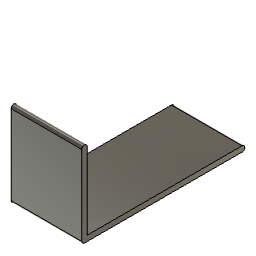
Nintendo 64 Bookends (Autodesk Fusion 360 design; units mm, degrees)
Autodesk Fusion 360 part; units mm, degrees
sketch "Sketch1" plane through (0, 0, 0) normal (0, 0, 1) x (1, 0, 0)
  line L0 (0, 0) -> (39, 0)
  line L1 (39, 0) -> (39, 87)
  line L2 (39, 87) -> (0, 87)
  line L3 (0, 87) -> (0, 0)
  line L4 (0, 0) -> (39, 0)
  line L5 (39, 0) -> (39, -3)
  line L6 (39, -3) -> (0, -3)
  line L7 (0, -3) -> (0, 0)
  dimension "d1" = 39
  dimension "d2" = 87
  dimension "d3" = 3
  constraint horizontal L0
  constraint vertical L1
  constraint horizontal L2
  constraint vertical L3
  constraint coincident L0.start L3.end
  constraint horizontal L4
  constraint vertical L5
  constraint horizontal L6
  constraint vertical L7
  measures "d1" distance of L0.start L0.end
  measures "d2" distance of L0.start L2.end
  measures "d3" distance of L0.start L6.end
extrude "Extrude1" add sketch "Sketch1" along normal blind 47 contours L0 L4 L5 L6 L7
extrude "Extrude2" add sketch "Sketch1" along normal blind 3 contours L0 L1 L2 L3 L4
fillet "Fillet1" radius 1.5 3 edges at (19.5, 87, 3) (19.5, 0, 47) (19.5, -3, 47)
fillet "Fillet2" radius 1.5 2 edges at (19.5, -3, 0) (19.5, 87, 0)
sketch "Sketch2" plane through (0, 0, 0) normal (0, 0, -1) x (1, 0, 0)
  line L0 (0, -85.5) -> (39, -85.5)
  line L1 (39, -85.5) -> (39, 1.5)
  line L2 (39, 1.5) -> (0, 1.5)
  line L3 (0, 1.5) -> (0, -85.5)
  line L4 (30.9966, -51.6762) -> (29.7025, -51.6762)
  line L5 (29.7025, -51.6762) -> (29.7025, -54.5517)
  line L6 (29.7025, -54.5517) -> (30.5781, -54.5517)
  line L7 (30.5781, -54.5517) -> (30.5781, -52.9028)
  line L8 (30.5781, -52.9028) -> (30.5856, -52.9028)
  line L9 (30.5856, -52.9028) -> (31.1629, -54.5517)
  line L10 (31.1629, -54.5517) -> (32.4569, -54.5517)
  line L11 (32.4569, -54.5517) -> (32.4569, -51.6762)
  line L12 (32.4569, -51.6762) -> (31.5818, -51.6762)
  line L13 (31.5818, -51.6762) -> (31.5818, -53.336)
  line L14 (31.5818, -53.336) -> (31.574, -53.336)
  line L15 (31.574, -53.336) -> (30.9966, -51.6762)
  line L16 (26.1146, -51.6762) -> (24.8204, -51.6762)
  line L17 (24.8204, -51.6762) -> (24.8204, -54.5517)
  line L18 (24.8204, -54.5517) -> (25.6956, -54.5517)
  line L19 (25.6956, -54.5517) -> (25.6956, -52.9028)
  line L20 (25.6956, -52.9028) -> (25.7034, -52.9028)
  line L21 (25.7034, -52.9028) -> (26.2807, -54.5517)
  line L22 (26.2807, -54.5517) -> (27.5748, -54.5517)
  line L23 (27.5748, -54.5517) -> (27.5748, -51.6762)
  line L24 (27.5748, -51.6762) -> (26.6994, -51.6762)
  line L25 (26.6994, -51.6762) -> (26.6994, -53.336)
  line L26 (26.6994, -53.336) -> (26.6918, -53.336)
  line L27 (26.6918, -53.336) -> (26.1146, -51.6762)
  line L28 (17.7082, -51.6762) -> (16.414, -51.6762)
  line L29 (16.414, -51.6762) -> (16.414, -54.5517)
  line L30 (16.414, -54.5517) -> (17.2893, -54.5517)
  line L31 (17.2893, -54.5517) -> (17.2893, -52.9028)
  line L32 (17.2893, -52.9028) -> (17.2972, -52.9028)
  line L33 (17.2972, -52.9028) -> (17.8744, -54.5517)
  line L34 (17.8744, -54.5517) -> (19.1685, -54.5517)
  line L35 (19.1685, -54.5517) -> (19.1685, -51.6762)
  line L36 (19.1685, -51.6762) -> (18.2934, -51.6762)
  line L37 (18.2934, -51.6762) -> (18.2934, -53.336)
  line L38 (18.2934, -53.336) -> (18.2857, -53.336)
  line L39 (18.2857, -53.336) -> (17.7082, -51.6762)
  line L40 (29.1739, -54.5517) -> (28.0946, -54.5517)
  line L41 (28.0946, -54.5517) -> (28.0946, -51.6762)
  line L42 (28.0946, -51.6762) -> (29.1739, -51.6762)
  line L43 (29.1739, -51.6762) -> (29.1739, -54.5517)
  line L44 (23.8216, -53.7705) -> (24.5075, -53.7705)
  line L45 (24.5075, -53.7705) -> (24.5075, -54.5517)
  line L46 (24.5075, -54.5517) -> (22.0544, -54.5517)
  line L47 (22.0544, -54.5517) -> (22.0544, -53.7705)
  line L48 (22.0544, -53.7705) -> (22.7426, -53.7705)
  line L49 (22.7426, -53.7705) -> (22.7426, -51.6762)
  line L50 (22.7426, -51.6762) -> (23.8216, -51.6762)
  line L51 (23.8216, -51.6762) -> (23.8216, -53.7705)
  line L52 (21.7356, -54.5524) -> (19.601, -54.5524)
  line L53 (19.601, -54.5524) -> (19.601, -53.7919)
  line L54 (19.601, -53.7919) -> (20.6733, -53.7919)
  line L55 (20.6733, -53.7919) -> (20.6733, -53.4911)
  line L56 (20.6733, -53.4911) -> (19.6859, -53.4911)
  line L57 (19.6859, -53.4911) -> (19.6859, -52.754)
  line L58 (19.6859, -52.754) -> (20.6733, -52.754)
  line L59 (20.6733, -52.754) -> (20.6733, -52.4313)
  line L60 (20.6733, -52.4313) -> (19.5669, -52.4313)
  line L61 (19.5669, -52.4313) -> (19.5669, -51.677)
  line L62 (19.5669, -51.677) -> (21.7356, -51.677)
  line L63 (21.7356, -51.677) -> (21.7356, -54.5524)
  line L64 (19.9291, -48.5819) -> (22.2174, -44.4981)
  line L65 (22.2174, -44.4981) -> (19.9291, -45.375)
  line L66 (19.9291, -45.375) -> (17.745, -44.5387)
  line L67 (17.745, -44.5387) -> (17.16, -45.1951)
  line L68 (17.16, -45.1951) -> (17.16, -49.6558)
  line L69 (17.16, -49.6558) -> (19.9291, -48.5819)
  line L70 (12.8202, -33.9096) -> (16.9532, -39.3035)
  line L71 (16.9532, -39.3035) -> (16.9532, -32.172)
  line L72 (16.9532, -32.172) -> (19.9292, -30.9133)
  line L73 (19.9292, -30.9133) -> (19.9292, -43.0951)
  line L74 (19.9292, -43.0951) -> (16.9532, -44.2347)
  line L75 (16.9532, -44.2347) -> (12.8202, -38.3275)
  line L76 (12.8202, -38.3275) -> (12.8202, -45.838)
  line L77 (12.8202, -45.838) -> (10.0098, -46.9218)
  line L78 (10.0098, -46.9218) -> (10.0098, -35.0899)
  line L79 (10.0098, -35.0899) -> (12.8202, -33.9096)
  line L80 (27.038, -33.9096) -> (24.4011, -35.0771)
  line L81 (24.4011, -35.0771) -> (27.038, -40.1964)
  line L82 (27.038, -40.1964) -> (27.038, -33.9096)
  line L83 (24.2275, -46.9219) -> (22.9048, -44.2351)
  line L84 (22.9048, -44.2351) -> (22.2174, -44.4981)
  line L85 (22.2174, -44.4981) -> (19.9291, -48.5819)
  line L86 (19.9291, -48.5819) -> (22.6984, -49.6589)
  line L87 (22.6984, -49.6589) -> (24.2275, -46.9219)
  line L88 (17.745, -44.5387) -> (15.6298, -46.9219)
  line L89 (15.6298, -46.9219) -> (12.8202, -45.838)
  line L90 (12.8202, -45.838) -> (12.8202, -38.3275)
  line L91 (12.8202, -38.3275) -> (16.9532, -44.2347)
  line L92 (16.9532, -44.2347) -> (17.745, -44.5387)
  line L93 (27.038, -45.8381) -> (29.8484, -46.9219)
  line L94 (29.8484, -46.9219) -> (29.8484, -35.09)
  line L95 (29.8484, -35.09) -> (27.038, -33.9096)
  line L96 (27.038, -33.9096) -> (27.038, -40.1964)
  line L97 (27.038, -40.1964) -> (22.9048, -32.1719)
  line L98 (22.9048, -32.1719) -> (19.9292, -30.9133)
  line L99 (19.9292, -30.9133) -> (19.9292, -43.0951)
  line L100 (19.9292, -43.0951) -> (22.9048, -44.2351)
  line L101 (22.9048, -44.2351) -> (22.9048, -38.0508)
  line L102 (22.9048, -38.0508) -> (27.038, -45.8381)
  line L103 (22.9048, -44.2351) -> (22.9048, -38.0508)
  line L104 (22.9048, -38.0508) -> (27.038, -45.8381)
  line L105 (27.038, -45.8381) -> (24.2275, -46.9219)
  line L106 (24.2275, -46.9219) -> (22.9048, -44.2351)
  line L107 (12.8202, -33.9096) -> (16.9532, -39.3035)
  line L108 (16.9532, -39.3035) -> (16.9532, -36.3566)
  line L109 (16.9532, -36.3566) -> (16.1092, -35.1726)
  line L110 (16.1092, -35.1726) -> (12.8202, -33.9096)
  line L111 (16.9532, -44.2347) -> (19.9292, -43.0951)
  line L112 (19.9292, -43.0951) -> (22.9048, -44.2351)
  line L113 (22.9048, -44.2351) -> (19.9291, -45.375)
  line L114 (19.9291, -45.375) -> (16.9532, -44.2347)
  line L115 (15.6308, -46.9219) -> (12.8202, -48.0031)
  line L116 (12.8202, -48.0031) -> (10.0098, -46.9218)
  line L117 (10.0098, -46.9218) -> (12.8202, -45.838)
  line L118 (12.8202, -45.838) -> (15.6308, -46.9219)
  line L119 (29.8484, -46.9219) -> (27.038, -48.0031)
  line L120 (27.038, -48.0031) -> (24.2275, -46.9219)
  line L121 (24.2275, -46.9219) -> (27.038, -45.8381)
  line L122 (27.038, -45.8381) -> (29.8484, -46.9219)
  line L123 (17.16, -49.6558) -> (19.9291, -50.725)
  line L124 (19.9291, -50.725) -> (22.6984, -49.6589)
  line L125 (22.6984, -49.6589) -> (19.9291, -48.5819)
  line L126 (19.9291, -48.5819) -> (17.16, -49.6558)
  line L127 (15.9488, -54.5521) -> (14.6703, -54.5521)
  spline S0 degree 3 poles (14.6703, -54.5521) (13.5786, -54.5521) (13.2338, -53.9344) (13.2338, -53.0833) knots 0 0 0 0 1 1 1 1
  spline S1 degree 3 poles (13.2338, -53.0833) (13.2338, -52.2322) (13.7689, -51.6756) (14.6056, -51.6756) knots 0 0 0 0 1 1 1 1
  line L128 (14.6056, -51.6756) -> (15.9487, -51.6756)
  line L129 (15.9487, -51.6756) -> (15.9488, -54.5521)
  line L130 (14.893, -52.3293) -> (14.7888, -52.3293)
  spline S2 degree 3 poles (14.7888, -52.3293) (14.6128, -52.3293) (14.4979, -52.3831) (14.4297, -52.4981) knots 0 0 0 0 1 1 1 1
  spline S3 degree 3 poles (14.4297, -52.4981) (14.3579, -52.6166) (14.3508, -52.8356) (14.3508, -53.1157) knots 0 0 0 0 1 1 1 1
  spline S4 degree 3 poles (14.3508, -53.1157) (14.3508, -53.3959) (14.358, -53.6113) (14.4297, -53.7298) knots 0 0 0 0 1 1 1 1
  spline S5 degree 3 poles (14.4297, -53.7298) (14.4979, -53.8447) (14.6129, -53.8986) (14.7888, -53.8986) knots 0 0 0 0 1 1 1 1
  line L131 (14.7888, -53.8986) -> (14.893, -53.8986)
  line L132 (14.893, -53.8986) -> (14.893, -52.3293)
  spline S6 degree 3 poles (11.5425, -54.6275) (10.6016, -54.6275) (10.1348, -54.0099) (10.1348, -53.1157) knots 0 0 0 0 1 1 1 1
  spline S7 degree 3 poles (10.1348, -53.1157) (10.1348, -52.2215) (10.6016, -51.6003) (11.5425, -51.6003) knots 0 0 0 0 1 1 1 1
  spline S8 degree 3 poles (11.5425, -51.6003) (12.4833, -51.6003) (12.9502, -52.2179) (12.9502, -53.1157) knots 0 0 0 0 1 1 1 1
  spline S9 degree 3 poles (12.9502, -53.1157) (12.9502, -54.0135) (12.4798, -54.6275) (11.5425, -54.6275) knots 0 0 0 0 1 1 1 1
  spline S10 degree 3 poles (11.5425, -52.3293) (11.3737, -52.3293) (11.2517, -52.4118) (11.2517, -53.1157) knots 0 0 0 0 1 1 1 1
  spline S11 degree 3 poles (11.2517, -53.1157) (11.2517, -53.8196) (11.3665, -53.8986) (11.5425, -53.8986) knots 0 0 0 0 1 1 1 1
  spline S12 degree 3 poles (11.5425, -53.8986) (11.7185, -53.8986) (11.8333, -53.8016) (11.8333, -53.1157) knots 0 0 0 0 1 1 1 1
  spline S13 degree 3 poles (11.8333, -53.1157) (11.8333, -52.4118) (11.7076, -52.3293) (11.5425, -52.3293) knots 0 0 0 0 1 1 1 1
  line L133 (30.9966, -51.6762) -> (29.7025, -51.6762)
  line L134 (29.7025, -51.6762) -> (29.7025, -54.5517)
  line L135 (29.7025, -54.5517) -> (30.5781, -54.5517)
  line L136 (30.5781, -54.5517) -> (30.5781, -52.9028)
  line L137 (30.5781, -52.9028) -> (30.5856, -52.9028)
  line L138 (30.5856, -52.9028) -> (31.1629, -54.5517)
  line L139 (31.1629, -54.5517) -> (32.4569, -54.5517)
  line L140 (32.4569, -54.5517) -> (32.4569, -51.6762)
  line L141 (32.4569, -51.6762) -> (31.5818, -51.6762)
  line L142 (31.5818, -51.6762) -> (31.5818, -53.336)
  line L143 (31.5818, -53.336) -> (31.574, -53.336)
  line L144 (31.574, -53.336) -> (30.9966, -51.6762)
  line L145 (26.1146, -51.6762) -> (24.8204, -51.6762)
  line L146 (24.8204, -51.6762) -> (24.8204, -54.5517)
  line L147 (24.8204, -54.5517) -> (25.6956, -54.5517)
  line L148 (25.6956, -54.5517) -> (25.6956, -52.9028)
  line L149 (25.6956, -52.9028) -> (25.7034, -52.9028)
  line L150 (25.7034, -52.9028) -> (26.2807, -54.5517)
  line L151 (26.2807, -54.5517) -> (27.5748, -54.5517)
  line L152 (27.5748, -54.5517) -> (27.5748, -51.6762)
  line L153 (27.5748, -51.6762) -> (26.6994, -51.6762)
  line L154 (26.6994, -51.6762) -> (26.6994, -53.336)
  line L155 (26.6994, -53.336) -> (26.6918, -53.336)
  line L156 (26.6918, -53.336) -> (26.1146, -51.6762)
  line L157 (17.7082, -51.6762) -> (16.414, -51.6762)
  line L158 (16.414, -51.6762) -> (16.414, -54.5517)
  line L159 (16.414, -54.5517) -> (17.2893, -54.5517)
  line L160 (17.2893, -54.5517) -> (17.2893, -52.9028)
  line L161 (17.2893, -52.9028) -> (17.2972, -52.9028)
  line L162 (17.2972, -52.9028) -> (17.8744, -54.5517)
  line L163 (17.8744, -54.5517) -> (19.1685, -54.5517)
  line L164 (19.1685, -54.5517) -> (19.1685, -51.6762)
  line L165 (19.1685, -51.6762) -> (18.2934, -51.6762)
  line L166 (18.2934, -51.6762) -> (18.2934, -53.336)
  line L167 (18.2934, -53.336) -> (18.2857, -53.336)
  line L168 (18.2857, -53.336) -> (17.7082, -51.6762)
  line L169 (29.1739, -54.5517) -> (28.0946, -54.5517)
  line L170 (28.0946, -54.5517) -> (28.0946, -51.6762)
  line L171 (28.0946, -51.6762) -> (29.1739, -51.6762)
  line L172 (29.1739, -51.6762) -> (29.1739, -54.5517)
  line L173 (23.8216, -53.7705) -> (24.5075, -53.7705)
  line L174 (24.5075, -53.7705) -> (24.5075, -54.5517)
  line L175 (24.5075, -54.5517) -> (22.0544, -54.5517)
  line L176 (22.0544, -54.5517) -> (22.0544, -53.7705)
  line L177 (22.0544, -53.7705) -> (22.7426, -53.7705)
  line L178 (22.7426, -53.7705) -> (22.7426, -51.6762)
  line L179 (22.7426, -51.6762) -> (23.8216, -51.6762)
  line L180 (23.8216, -51.6762) -> (23.8216, -53.7705)
  line L181 (21.7356, -54.5524) -> (19.601, -54.5524)
  line L182 (19.601, -54.5524) -> (19.601, -53.7919)
  line L183 (19.601, -53.7919) -> (20.6733, -53.7919)
  line L184 (20.6733, -53.7919) -> (20.6733, -53.4911)
  line L185 (20.6733, -53.4911) -> (19.6859, -53.4911)
  line L186 (19.6859, -53.4911) -> (19.6859, -52.754)
  line L187 (19.6859, -52.754) -> (20.6733, -52.754)
  line L188 (20.6733, -52.754) -> (20.6733, -52.4313)
  line L189 (20.6733, -52.4313) -> (19.5669, -52.4313)
  line L190 (19.5669, -52.4313) -> (19.5669, -51.677)
  line L191 (19.5669, -51.677) -> (21.7356, -51.677)
  line L192 (21.7356, -51.677) -> (21.7356, -54.5524)
  spline S14 degree 3 poles (8.2028, -54.9328) (8.2603, -54.94) (8.3178, -54.9364) (8.3931, -54.9328) knots 0 0 0 0 1 1 1 1
  spline S15 degree 3 poles (8.3931, -54.9328) (8.8491, -54.9112) (9.0323, -54.7173) (9.097, -54.4982) knots 0 0 0 0 1 1 1 1
  line L193 (9.097, -54.4982) -> (9.0862, -54.4982)
  spline S16 degree 3 poles (9.0862, -54.4982) (8.9714, -54.5988) (8.8313, -54.6454) (8.6445, -54.6454) knots 0 0 0 0 1 1 1 1
  spline S17 degree 3 poles (8.6445, -54.6454) (8.2818, -54.6454) (7.955, -54.3833) (7.955, -53.8877) knots 0 0 0 0 1 1 1 1
  spline S18 degree 3 poles (7.955, -53.8877) (7.955, -53.392) (8.314, -53.0509) (8.8025, -53.0509) knots 0 0 0 0 1 1 1 1
  spline S19 degree 3 poles (8.8025, -53.0509) (9.4417, -53.0509) (9.7217, -53.5394) (9.7217, -54.0637) knots 0 0 0 0 1 1 1 1
  spline S20 degree 3 poles (9.7217, -54.0637) (9.7217, -54.491) (9.5709, -54.8501) (9.3232, -55.0836) knots 0 0 0 0 1 1 1 1
  spline S21 degree 3 poles (9.3232, -55.0836) (9.0861, -55.3027) (8.7809, -55.414) (8.4074, -55.4211) knots 0 0 0 0 1 1 1 1
  spline S22 degree 3 poles (8.4074, -55.4211) (8.3105, -55.4283) (8.2494, -55.4211) (8.2027, -55.4175) knots 0 0 0 0 1 1 1 1
  line L194 (8.2027, -55.4175) -> (8.2028, -54.9328)
  spline S23 degree 3 poles (8.8097, -53.5143) (8.6623, -53.5143) (8.5726, -53.6651) (8.5726, -53.859) knots 0 0 0 0 1 1 1 1
  spline S24 degree 3 poles (8.5726, -53.859) (8.5726, -54.0206) (8.6481, -54.1966) (8.8455, -54.1966) knots 0 0 0 0 1 1 1 1
  spline S25 degree 3 poles (8.8455, -54.1966) (8.9676, -54.1966) (9.061, -54.1211) (9.0969, -54.0278) knots 0 0 0 0 1 1 1 1
  spline S26 degree 3 poles (9.0969, -54.0278) (9.1112, -53.9991) (9.1149, -53.9596) (9.1149, -53.8914) knots 0 0 0 0 1 1 1 1
  spline S27 degree 3 poles (9.1149, -53.8914) (9.1041, -53.7082) (9.0143, -53.5143) (8.8133, -53.5143) knots 0 0 0 0 1 1 1 1
  line L195 (8.8133, -53.5143) -> (8.8097, -53.5143)
  line L196 (6.8238, -53.0905) -> (6.8238, -53.604)
  line L197 (6.8238, -53.604) -> (7.7827, -53.604)
  line L198 (7.7827, -53.604) -> (7.7827, -54.017)
  line L199 (7.7827, -54.017) -> (7.0141, -55.3888)
  line L200 (7.0141, -55.3888) -> (6.2456, -55.3888)
  line L201 (6.2456, -55.3888) -> (6.2456, -54.0781)
  line L202 (6.2456, -54.0781) -> (6.0015, -54.0781)
  line L203 (6.0015, -54.0781) -> (6.0015, -53.604)
  line L204 (6.0015, -53.604) -> (6.2456, -53.604)
  line L205 (6.2456, -53.604) -> (6.2456, -53.0905)
  line L206 (6.2456, -53.0905) -> (6.8238, -53.0905)
  line L207 (6.8238, -54.0781) -> (6.8238, -54.473)
  spline S28 degree 3 poles (6.8238, -54.473) (6.8238, -54.6202) (6.8166, -54.7711) (6.8095, -54.9327) knots 0 0 0 0 1 1 1 1
  line L208 (6.8095, -54.9327) -> (6.8203, -54.9327)
  spline S29 degree 3 poles (6.8203, -54.9327) (6.8922, -54.7747) (6.9531, -54.6274) (7.0358, -54.4694) knots 0 0 0 0 1 1 1 1
  line L209 (7.0358, -54.4694) -> (7.2225, -54.0851)
  line L210 (7.2225, -54.0851) -> (7.2261, -54.078)
  line L211 (7.2261, -54.078) -> (6.8238, -54.0781)
extrude "Extrude3" cut sketch "Sketch2" against normal blind 1 contours L4 L5 L6 L7 L8 L9 L10 L11 L12 L13 L14 L15 L133 L134 L135 L136 L137 L138 L139 L140 L141 L142 L143 L144 | L16 L17 L18 L19 L20 L21 L22 L23 L24 L25 L26 L27 L145 L146 L147 L148 L149 L150 L151 L152 L153 L154 L155 L156 | L28 L29 L30 L31 L32 L33 L34 L35 L36 L37 L38 L39 L157 L158 L159 L160 L161 L162 L163 L164 L165 L166 L167 L168 | L40 L41 L42 L43 L169 L170 L171 L172 | L44 L45 L46 L47 L48 L49 L50 L51 L173 L174 L175 L176 L177 L178 L179 L180 | L52 L53 L54 L55 L56 L57 L58 L59 L60 L61 L62 L63 L181 L182 L183 L184 L185 L186 L187 L188 L189 L190 L191 L192 | L127 S0 S1 L128 L129 | S6 S7 S8 S9 | S14 S15 L193 S16 S17 S18 S19 S20 S21 S22 L194 | L196 L197 L198 L199 L200 L201 L202 L203 L204 L205 L206
extrude "Extrude4" cut sketch "Sketch2" against normal blind 1 contours L73 L81 L82 L93 L94 L95 L96 L97 L98 L99 L100 L101 L102 L103 L104 L112 L122
extrude "Extrude5" cut sketch "Sketch2" against normal blind 0.5 contours L70 L71 L72 L73 L74 L75 L76 L77 L78 L79 L90 L91 L99 L107 L108 L111 L117
